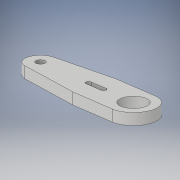
# Autodesk Inventor part: 小零件5
Saved by Autodesk Inventor 2017 (Build 210142000, 142)
## iProperties
Part Number: 小零件5
Material: 一般
Document SubType Name: Modeling
Designer: User
Density: 1 g/cm^3
Appearance: 預設
Author: User
Autodesk Inventor part; units mm, degrees
ref_plane "YZ Plane" through (0, 0, 0) normal (1, 0, 0) x (0, 1, 0)
ref_plane "XZ Plane" through (0, 0, 0) normal (0, 1, 0) x (-1, 0, 0)
ref_plane "XY Plane" through (0, 0, 0) normal (0, 0, 1) x (1, 0, 0)
sketch "草圖1" plane through (0, 0, 0) normal (0, 1, 0) x (-1, 0, 0)
  circle A0 centre (0, 0) radius 1.25
  arc A1 (0.4393, -3.9758) -> (0.4393, 3.9758) centre (0, 0) ccw
  arc A2 (-31, 6) -> (-31, -6) centre (-31, 0) ccw
  circle A3 centre (-31, 0) radius 3.6
  line L0 (-31, 0) -> (-31, -6)
  line L1 (-31, -6) -> (-17.88, -6)
  line L2 (-17.88, -6) -> (0.4393, -3.9758)
  line L3 (-21, 0) -> (-16, 0) construction
  line L4 (-21, -0.75) -> (-16, -0.75)
  line L5 (-16, 0.75) -> (-21, 0.75)
  arc A4 (-21, 0.75) -> (-21, -0.75) centre (-21, 0) ccw
  arc A5 (-16, -0.75) -> (-16, 0.75) centre (-16, 0) ccw
  line L6 (-31, 6) -> (-17.88, 6)
  line L7 (-17.88, 6) -> (0.4393, 3.9758)
  point P0 (-18.5, 0)
  dimension "d0" = 2.5
  dimension "d1" = 8
  dimension "d3" = 12
  dimension "d4" = 7.2
  dimension "d5" = 13.12
  dimension "d6" = 10
  dimension "d7" = 5
  dimension "d8" = 1.5
  constraints: 18 end point, 8 point on circle, 6 centre point, 5 tangent, 3 coincident, 1 midpoint, 1 parallel, 1 perpendicular, 1 vertical
  measures "d0" diameter of A0
  measures "d1" diameter of A1
  measures "d3" diameter of A2
  measures "d4" diameter of A3
  measures "d5" distance of L0.end L1.end
  measures "d6" distance of L0.start L3.start
  measures "d7" distance of L3.start L3.end
  measures "d8" diameter of A5
extrude "擠出1" add sketch "草圖1" along normal mid plane 3
